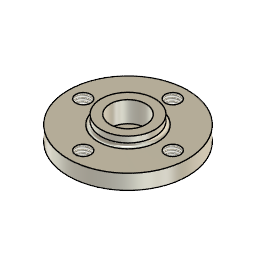
ServoHorn_v1 (Autodesk Fusion 360 design; units mm, degrees)
Autodesk Fusion 360 part; units mm, degrees
sketch "Sketch1" plane through (0, 0, 0) normal (0, 0, 1) x (1, 0, 0)
  circle A0 centre (0, 0) radius 10
  circle A1 centre (0, 0) radius 7.5 construction
  circle A2 centre (0, 7.5) radius 1.5
  circle A3 centre (-7.5, 0) radius 1.5
  circle A4 centre (0, -7.5) radius 1.5
  circle A5 centre (7.5, 0) radius 1.5
  line L0 (0, 7.5) -> (0, 0) construction
  circle A6 centre (0, 0) radius 4.5
  circle A7 centre (0, 0) radius 1.6
  circle A8 centre (0, 0) radius 3
  dimension "d1" = 20
  dimension "d2" = 15
  dimension "d3" = 3
  dimension "d6" = 360
  dimension "d7" = 9
  dimension "d8" = 3.2
  dimension "d9" = 6
  constraint coincident A0.centre A1.centre
  constraint coincident A1 A2.centre
  constraint coincident A2.centre L0.start
  constraint vertical L0
  constraint concentric A1 A6
  constraint concentric A0 A8
  measures "d1" diameter of A0
  measures "d2" diameter of A1
  measures "d3" diameter of A2
  measures "d7" diameter of A6
  measures "d8" diameter of A7
  measures "d9" diameter of A8
extrude "Extrude1" add sketch "Sketch1" against normal blind 2.5 contours A0 | A6 | A8
extrude "Extrude2" add sketch "Sketch1" along normal blind 1.5 contours A6
fillet "Fillet1" radius 0.5 1 edges at (-4.1955, 1.6273, 0)
move_face "OffsetFaces1" offset -2 1 faces at (2.5162, -0.2285, 0)
thread "Thread1" "ISO Metric profile 3.0 M3x0.5 M3x0.5 6H" major diameter 3.086 minor diameter 2.529 pitch 0.5 angle 60 resizes the face on face at (1.4981, -7.5748, -1.6667) on face at (-6.0019, -0.0748, -1.6667) on face at (8.9981, -0.0748, -1.6667) on face at (1.4981, 7.4252, -1.6667)
